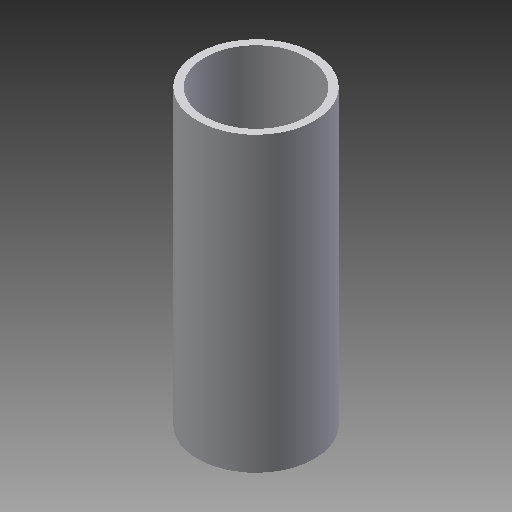
# Autodesk Inventor part: Rura_pionowa_kolka_rzedniego
Saved by Autodesk Inventor 2017 (Build 210142000, 142)
## iProperties
Created: 2015-11-22
Part Number: Rura_pionowa_kolka_rzedniego
Material: Aluminium AW-7020
Document SubType Name: Modeling
Designer: graaapsik
Density: 2.78 g/cm^3
Appearance: Aluminium AW-7020
Mass: 41.9214 g
Surface Area: 154.566 cm^2
Volume: 15.0796 cm^3
Author: graaapsik
Autodesk Inventor part; units mm, degrees
ref_plane "YZ Plane" through (0, 0, 0) normal (1, 0, 0) x (0, 1, 0)
ref_plane "XZ Plane" through (0, 0, 0) normal (0, 1, 0) x (-1, 0, 0)
ref_plane "XY Plane" through (0, 0, 0) normal (0, 0, 1) x (1, 0, 0)
sketch "Szkic1" plane through (0, 0, 0) normal (0, 1, 0) x (-1, 0, 0)
  circle A0 centre (0, 0) radius 16
  dimension "d0" = 32
  constraints: 1 centre point, 1 coincident
  measures "d0" diameter of A0
extrude "Wyciągnięcie proste1" add sketch "Szkic1" along normal blind 80
shell "Skorupa1" thickness 2 removed faces 2 at (-4.7224, 0, 2.4785) at (-4.7224, 80, 2.4785)
